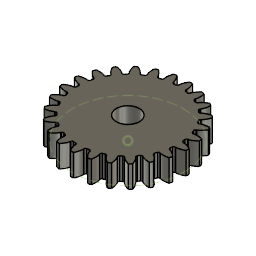
Third gear (Autodesk Fusion 360 design; units mm, degrees)
part number: 2026-05-25-19-30-06-242
Autodesk Fusion 360 part; units mm, degrees
sketch "Base Circle" plane through (0, 0, 0) normal (0, 0, 1) x (1, 0, 0)
  circle A0 centre (0, 0) radius 11.343
  circle A1 centre (0, 0) radius 2.6
extrude "Extrude1" add sketch "Base Circle" along normal blind 5
sketch "Gear Tooth" plane through (0, 0, 0) normal (0, 0, 1) x (1, 0, 0)
  spline S0 degree 5 poles (11.7116, -0.9005) (11.7167, -0.9009) (11.7269, -0.9015) (11.7422, -0.9021) (11.7626, -0.9022) (11.7882, -0.9014) (11.8137, -0.8998) (11.8394, -0.8977) (11.865, -0.8955) (11.8906, -0.893) (11.9163, -0.8904) (11.9419, -0.8876) (11.9676, -0.8845) (11.9933, -0.8811) (12.0189, -0.8773) (12.0446, -0.8732) (12.0703, -0.8688) (12.096, -0.8641) (12.1216, -0.8593) (12.1473, -0.8543) (12.173, -0.8491) (12.1987, -0.8437) (12.2244, -0.838) (12.25, -0.8322) (12.2757, -0.8262) (12.3014, -0.8199) (12.3271, -0.8135) (12.3527, -0.8068) (12.3784, -0.8) (12.404, -0.793) (12.4297, -0.7859) (12.4553, -0.7785) (12.4809, -0.771) (12.5066, -0.7633) (12.5322, -0.7555) (12.5578, -0.7475) (12.5834, -0.7393) (12.609, -0.7309) (12.6345, -0.7224) (12.6601, -0.7137) (12.6857, -0.7049) (12.7112, -0.6959) (12.7367, -0.6868) (12.7623, -0.6775) (12.7878, -0.668) (12.8133, -0.6584) (12.8387, -0.6487) (12.8642, -0.6388) (12.8897, -0.6287) (12.9151, -0.6185) (12.9405, -0.6082) (12.9659, -0.5977) (12.9913, -0.5871) (13.0167, -0.5764) (13.0421, -0.5655) (13.0674, -0.5544) (13.0928, -0.5433) (13.1181, -0.532) (13.1434, -0.5205) (13.1687, -0.5089) (13.1939, -0.4972) (13.2192, -0.4854) (13.2444, -0.4734) (13.2696, -0.4613) (13.2948, -0.449) (13.32, -0.4366) (13.3451, -0.4241) (13.3702, -0.4115) (13.3953, -0.3987) (13.4204, -0.3858) (13.4455, -0.3728) (13.4655, -0.3623) (13.4805, -0.3544) (13.4906, -0.349) (13.4956, -0.3464) knots 0 0 0 0 0 0 0.01428571 0.02857143 0.04285714 0.05714286 0.07142857 0.08571429 0.1 0.11428571 0.12857143 0.14285714 0.15714286 0.17142857 0.18571429 0.2 0.21428571 0.22857143 0.24285714 0.25714286 0.27142857 0.28571429 0.3 0.31428571 0.32857143 0.34285714 0.35714286 0.37142857 0.38571429 0.4 0.41428571 0.42857143 0.44285714 0.45714286 0.47142857 0.48571429 0.5 0.51428571 0.52857143 0.54285714 0.55714286 0.57142857 0.58571429 0.6 0.61428571 0.62857143 0.64285714 0.65714286 0.67142857 0.68571429 0.7 0.71428571 0.72857143 0.74285714 0.75714286 0.77142857 0.78571429 0.8 0.81428571 0.82857143 0.84285714 0.85714286 0.87142857 0.88571429 0.9 0.91428571 0.92857143 0.94285714 0.95714286 0.97142857 0.98571429 1 1 1 1 1 1
  spline S1 degree 5 poles (11.7116, 0.9005) (11.7167, 0.9009) (11.7269, 0.9015) (11.7422, 0.9021) (11.7626, 0.9022) (11.7882, 0.9014) (11.8137, 0.8998) (11.8394, 0.8977) (11.865, 0.8955) (11.8906, 0.893) (11.9163, 0.8904) (11.9419, 0.8876) (11.9676, 0.8845) (11.9933, 0.8811) (12.0189, 0.8773) (12.0446, 0.8732) (12.0703, 0.8688) (12.096, 0.8641) (12.1216, 0.8593) (12.1473, 0.8543) (12.173, 0.8491) (12.1987, 0.8437) (12.2244, 0.838) (12.25, 0.8322) (12.2757, 0.8262) (12.3014, 0.8199) (12.3271, 0.8135) (12.3527, 0.8068) (12.3784, 0.8) (12.404, 0.793) (12.4297, 0.7859) (12.4553, 0.7785) (12.4809, 0.771) (12.5066, 0.7633) (12.5322, 0.7555) (12.5578, 0.7475) (12.5834, 0.7393) (12.609, 0.7309) (12.6345, 0.7224) (12.6601, 0.7137) (12.6857, 0.7049) (12.7112, 0.6959) (12.7367, 0.6868) (12.7623, 0.6775) (12.7878, 0.668) (12.8133, 0.6584) (12.8387, 0.6487) (12.8642, 0.6388) (12.8897, 0.6287) (12.9151, 0.6185) (12.9405, 0.6082) (12.9659, 0.5977) (12.9913, 0.5871) (13.0167, 0.5764) (13.0421, 0.5655) (13.0674, 0.5544) (13.0928, 0.5433) (13.1181, 0.532) (13.1434, 0.5205) (13.1687, 0.5089) (13.1939, 0.4972) (13.2192, 0.4854) (13.2444, 0.4734) (13.2696, 0.4613) (13.2948, 0.449) (13.32, 0.4366) (13.3451, 0.4241) (13.3702, 0.4115) (13.3953, 0.3987) (13.4204, 0.3858) (13.4455, 0.3728) (13.4655, 0.3623) (13.4805, 0.3544) (13.4906, 0.349) (13.4956, 0.3464) knots 0 0 0 0 0 0 0.01428571 0.02857143 0.04285714 0.05714286 0.07142857 0.08571429 0.1 0.11428571 0.12857143 0.14285714 0.15714286 0.17142857 0.18571429 0.2 0.21428571 0.22857143 0.24285714 0.25714286 0.27142857 0.28571429 0.3 0.31428571 0.32857143 0.34285714 0.35714286 0.37142857 0.38571429 0.4 0.41428571 0.42857143 0.44285714 0.45714286 0.47142857 0.48571429 0.5 0.51428571 0.52857143 0.54285714 0.55714286 0.57142857 0.58571429 0.6 0.61428571 0.62857143 0.64285714 0.65714286 0.67142857 0.68571429 0.7 0.71428571 0.72857143 0.74285714 0.75714286 0.77142857 0.78571429 0.8 0.81428571 0.82857143 0.84285714 0.85714286 0.87142857 0.88571429 0.9 0.91428571 0.92857143 0.94285714 0.95714286 0.97142857 0.98571429 1 1 1 1 1 1
  arc A0 (13.4956, -0.3464) -> (13.4956, 0.3464) centre (0, 0) ccw
  line L0 (11.2996, -0.8688) -> (11.7116, -0.9005)
  line L1 (11.2996, 0.8688) -> (11.7116, 0.9005)
  line L2 (11.2996, -0.8688) -> (11.2996, 0.8688)
  point P0 (11.8374, -0.8978)
  point P1 (11.964, -0.8849)
  point P2 (12.0911, -0.865)
  point P3 (12.2185, -0.8393)
  point P4 (12.3461, -0.8085)
  point P5 (12.4739, -0.7731)
  point P6 (12.6018, -0.7332)
  point P7 (12.7297, -0.6892)
  point P8 (12.8576, -0.6413)
  point P9 (12.9855, -0.5895)
  point P10 (13.1133, -0.5341)
  point P11 (13.2409, -0.475)
  point P12 (13.3684, -0.4124)
  point P13 (11.8374, 0.8978)
  point P14 (11.964, 0.8849)
  point P15 (12.0911, 0.865)
  point P16 (12.2185, 0.8393)
  point P17 (12.3461, 0.8085)
  point P18 (12.4739, 0.7731)
  point P19 (12.6018, 0.7332)
  point P20 (12.7297, 0.6892)
  point P21 (12.8576, 0.6413)
  point P22 (12.9855, 0.5895)
  point P23 (13.1133, 0.5341)
  point P24 (13.2409, 0.475)
  point P25 (13.3684, 0.4124)
extrude "Extrude2" add sketch "Gear Tooth" along normal blind 5
fillet "Fillet1" radius 0.3 2 edges at (11.3096, -0.8696, 2.5) (11.3096, 0.8696, 2.5)
pattern_circular "C-Pattern1" count 25 over 360 about axis through (0, 0, 0) along (0, 0, 1) of "Extrude2", "Fillet1"
sketch "Diametrial Pitch Circle" plane through (0, 0, 0) normal (0, 0, 1) x (1, 0, 0)
  circle A0 centre (0, 0) radius 12.5 construction
named bodies: "Spur Gear (25 teeth)"
